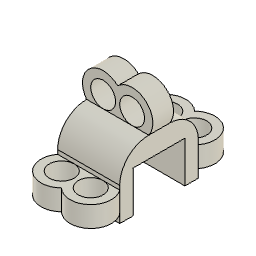
cleaning_cartridge_bracket v4 (Autodesk Fusion 360 design; units mm, degrees)
Autodesk Fusion 360 part; units mm, degrees
note: some values were not read from the file. Set by a fixed rule: which sketch regions a step uses.
sketch "Sketch1" plane through (0, 0, 0) normal (0, 0, 1) x (1, 0, 0)
  line L0 (7.5, -9.5) -> (-7.5, -9.5)
  line L1 (-7.5, -9.5) -> (-7.5, 9.5)
  line L2 (-7.5, 9.5) -> (7.5, 9.5)
  line L3 (7.5, 9.5) -> (7.5, -9.5)
  line L4 (7.5, -9.5) -> (-7.5, 9.5) construction
  line L5 (-7.5, -9.5) -> (7.5, 9.5) construction
  dimension "d1" = 15
  dimension "d2" = 19
  constraint horizontal L0
  constraint perpendicular L0 L1
  constraint parallel L0 L2
  constraint parallel L1 L3
  constraint coincident L4 origin
  constraint coincident L5 origin
  measures "d1" distance of L1.end L2.end
  measures "d2" distance of L0.end L1.end
extrude "Extrude1" add sketch "Sketch1" against normal blind 15
sketch "Sketch2" plane through (0, 0, -15) normal (0, 0, -1) x (1, 0, 0)
  line L0 (-7.5, -9.5) -> (7.5, -9.5)
  line L1 (7.5, -9.5) -> (7.5, 9.5)
  line L2 (7.5, 9.5) -> (-7.5, 9.5)
  line L3 (-7.5, 9.5) -> (-7.5, -9.5)
  line L4 (7.5, 6.25) -> (-7.5, 6.25)
  line L5 (-7.5, 6.25) -> (-7.5, -6.25)
  line L6 (-7.5, -6.25) -> (7.5, -6.25)
  line L7 (7.5, -6.25) -> (7.5, 6.25)
  line L8 (7.5, 6.25) -> (-7.5, -6.25) construction
  line L9 (-7.5, 6.25) -> (7.5, -6.25) construction
  dimension "d5" = 15
  dimension "d6" = 12.5
  constraint horizontal L4
  constraint perpendicular L4 L5
  constraint parallel L4 L6
  constraint parallel L5 L7
  constraint coincident L8 origin
  constraint coincident L9 origin
  measures "d5" distance of L5.end L6.end
  measures "d6" distance of L4.end L5.end
extrude "Extrude2" cut sketch "Sketch2" against normal blind 10 contours L1 L3 L4 L5 L6 L7
fillet "Fillet1" radius 7 2 edges at (0, 9.5, 0) (0, -9.5, 0)
ref_plane "WorkPlane1" through (0, 0, 0) normal (0, 1, 0) x (0, 0, 1)
sketch "Sketch4" plane through (0, 0, 0) normal (0, 1, 0) x (1, 0, 0)
  line L0 (-7.5, 0) -> (-7.5, 7)
  line L1 (7.5, 7) -> (7.5, 0)
  line L2 (7.5, 0) -> (-7.5, 0)
  line L3 (-7.5, 7) -> (-7.5, 15)
  line L4 (7.5, 15) -> (-7.5, 15)
  line L5 (7.5, 7) -> (7.5, 15)
  line L6 (0, 0) -> (-3.5, 0) construction
  line L7 (0, 0) -> (3.5, 0) construction
  line L8 (-3.5, 0) -> (-3.5, -3) construction
  line L9 (3.5, 0) -> (3.5, -3) construction
  circle A0 centre (3.5, -3) radius 3
  circle A1 centre (-3.5, -3) radius 3
  circle A2 centre (-3.5, -3) radius 5
  circle A3 centre (3.5, -3) radius 5
  dimension "d20" = 3.5
  dimension "d21" = 3.5
  dimension "d22" = 3
  dimension "d23" = 3
  dimension "d24" = 6
  dimension "d25" = 6
  dimension "d26" = 10
  dimension "d27" = 10
  constraint coincident L6.start L7.start
  constraint parallel L2 L6
  constraint parallel L2 L7
  constraint perpendicular L2 L8
  constraint perpendicular L7 L9
  constraint coincident L9.end A0.centre
  constraint coincident L8.end A1.centre
  constraint concentric A1 A2
  constraint concentric A0 A3
  measures "d20" distance of L6.start L6.end
  measures "d21" distance of L6.start L7.end
  measures "d22" distance of L6.end L8.end
  measures "d23" distance of L7.end L9.end
  measures "d24" diameter of A0
  measures "d25" diameter of A1
  measures "d26" diameter of A2
  measures "d27" diameter of A3
extrude "Extrude3" add sketch "Sketch4" along normal mid plane 5 contours L2 A2 A3 | L2 A1 A2 A3 | L2 A1 A3 | L2 A2 A3 | L2 A0 A1 A2 A3 | L2 A0 A2 A3 | L2 A0 A2 picked at (-1.7132, 0.4693) picked at (1.7132, 0.4693)
ref_plane "WorkPlane2" through (0, 0, -8) normal (0, 0, 1) x (1, 0, 0)
sketch "Sketch5" plane through (0, 0, -8) normal (0, 0, 1) x (1, 0, 0)
  line L0 (-7.5, 6.25) -> (-7.5, 9.5)
  line L1 (-7.5, -9.5) -> (-7.5, -6.25)
  line L2 (-7.5, 9.5) -> (7.5, 9.5)
  line L3 (7.5, 9.5) -> (7.5, 6.25)
  line L4 (7.5, -6.25) -> (7.5, -9.5)
  line L5 (7.5, -9.5) -> (-7.5, -9.5)
  line L6 (0, 9.5) -> (-3.5, 9.5) construction
  line L7 (0, 9.5) -> (3.5, 9.5) construction
  line L8 (-3.5, 9.5) -> (-3.5, 12.5) construction
  line L9 (3.5, 9.5) -> (3.5, 12.5) construction
  line L10 (10.0516, 0) -> (-10.1091, 0) construction
  circle A0 centre (3.5, 12.5) radius 3
  circle A1 centre (-3.5, 12.5) radius 3
  circle A2 centre (-3.5, 12.5) radius 5
  circle A3 centre (3.5, 12.5) radius 5
  circle A4 centre (3.5, -12.5) radius 5
  circle A5 centre (3.5, -12.5) radius 3
  circle A6 centre (-3.5, -12.5) radius 5
  circle A7 centre (-3.5, -12.5) radius 3
  line L11 (8.5, 2.5) -> (7.5, 2.5)
  line L12 (7.5, -2.5) -> (8.5, -2.5)
  line L13 (7.5, -6.25) -> (7.5, -2.5)
  line L14 (7.5, 2.5) -> (7.5, 6.25)
  line L15 (8.5, 2.5) -> (8.5, -2.5)
  line L16 (-7.5, 2.5) -> (-8.5, 2.5)
  line L17 (-8.5, -2.5) -> (-7.5, -2.5)
  line L18 (-7.5, 6.25) -> (-7.5, 2.5)
  line L19 (-7.5, -2.5) -> (-7.5, -6.25)
  line L20 (-8.5, 2.5) -> (-8.5, -2.5)
  dimension "d31" = 3.5
  dimension "d32" = 3.5
  dimension "d33" = 3
  dimension "d34" = 3
  dimension "d35" = 6
  dimension "d36" = 6
  dimension "d37" = 10
  dimension "d38" = 10
  constraint midpoint L2 L6.start
  constraint perpendicular L0 L6
  constraint parallel L2 L7
  constraint perpendicular L6 L8
  constraint perpendicular L7 L9
  constraint coincident L9.end A0.centre
  constraint coincident L8.end A1.centre
  constraint concentric A1 A2
  constraint concentric A0 A3
  constraint symmetric L10 A0 A5
  constraint symmetric L10 A1 A7
  constraint symmetric L10 A2 A6
  constraint symmetric L10 A3 A4
  measures "d31" distance of L6.start L6.end
  measures "d32" distance of L6.start L7.end
  measures "d33" distance of L6.end L8.end
  measures "d34" distance of L7.end L9.end
  measures "d35" diameter of A0
  measures "d36" diameter of A1
  measures "d37" diameter of A2
  measures "d38" diameter of A3
extrude "Extrude4" add sketch "Sketch5" against normal blind 5 contours L2 A1 A2 A3 | L2 A1 A3 | L2 A0 A2 A3 | L2 A0 A1 A2 A3 | L2 A0 A2 | L5 A4 A6 A7 | L5 A4 A7 | L5 A4 A5 A6 | L5 A4 A5 A6 A7 | L5 A5 A6
equation "d2 = 13 mm + 3 mm + 3 mm"
